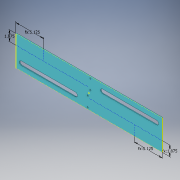
# Autodesk Inventor part: 5.5 x 27 x 1/8 x 3/8
Saved by Autodesk Inventor 2016 (Build 200138000, 138)
## iProperties
Created: 2015-06-18
Part Number: 5.5 x 27 x 1/8 x 3/8
Material: Aluminum 6061
Document SubType Name: Modeling
Designer: steele
Density: 2.7 g/cm^3
Appearance: Cadet Blue
Mass: 732.367 g
Surface Area: 1799.65 cm^2
Volume: 271.247 cm^3
Author: steele
Autodesk Inventor part; units mm, degrees
ref_plane "YZ Plane" through (0, 0, 0) normal (1, 0, 0) x (0, 1, 0)
ref_plane "XZ Plane" through (0, 0, 0) normal (0, 1, 0) x (-1, 0, 0)
ref_plane "XY Plane" through (0, 0, 0) normal (0, 0, 1) x (1, 0, 0)
sketch "Sketch1" plane through (0, 0, 0) normal (1, 0, 0) x (0, 1, 0)
  line L0 (-69.85, 342.9) -> (-69.85, -342.9)
  line L1 (-69.85, -342.9) -> (69.85, -342.9)
  line L2 (69.85, -342.9) -> (69.85, 342.9)
  line L3 (69.85, 342.9) -> (-69.85, 342.9)
  line L4 (-69.85, 342.9) -> (69.85, -342.9) construction
  line L5 (-69.85, -342.9) -> (69.85, 342.9) construction
  point P0 (0, 0)
  dimension "width" = 685.8
  dimension "height" = 139.7
  constraints: 12 end point, 2 midpoint, 2 parallel, 1 perpendicular, 1 vertical
  measures "width" distance of L0.start L0.end
  measures "height" distance of L0.end L1.end
extrude "Extrusion1" add sketch "Sketch1" along normal blind 3.175
sketch "Sketch2" plane through (3.175, 0, 0) normal (1, 0, 0) x (0, 0, -1)
  line L0 (-317.5, 38.1) -> (-63.5, 38.1) construction
  line L1 (-317.5, 28.575) -> (-63.5, 28.575)
  line L2 (-63.5, 47.625) -> (-317.5, 47.625)
  arc A0 (-317.5, 47.625) -> (-317.5, 28.575) centre (-317.5, 38.1) ccw
  arc A1 (-63.5, 28.575) -> (-63.5, 47.625) centre (-63.5, 38.1) ccw
  line L3 (342.9, 69.85) -> (-342.9, 69.85) projected
  line L4 (-342.9, 69.85) -> (-342.9, -69.85) projected
  line L5 (63.5, -38.1) -> (317.5, -38.1) construction
  line L6 (63.5, -47.625) -> (317.5, -47.625)
  line L7 (317.5, -28.575) -> (63.5, -28.575)
  arc A2 (63.5, -28.575) -> (63.5, -47.625) centre (63.5, -38.1) ccw
  arc A3 (317.5, -47.625) -> (317.5, -28.575) centre (317.5, -38.1) ccw
  line L8 (-342.9, -69.85) -> (342.9, -69.85) projected
  line L9 (342.9, -69.85) -> (342.9, 69.85) projected
  point P0 (0, 0)
  point P1 (-190.5, 38.1)
  point P2 (190.5, -38.1)
  dimension "slot_center_from_top" = 31.75
  dimension "slot_center_from_side" = 152.4
  dimension "slot_radius" = 9.525
  dimension "d7" = 31.75
  dimension "d8" = 152.4
  dimension "d9" = 9.525
  dimension "length_of_slot" = 254
  dimension "d13" = 254
  constraints: 16 end point, 8 point on circle, 8 tangent, 4 centre point, 2 horizontal, 2 midpoint, 2 parallel
  measures "slot_center_from_top" distance from line of point (-190.5, 38.1) L3
  measures "slot_center_from_side" distance from line of point (-190.5, 38.1) L4
  measures "slot_radius" radius of A1
  measures "d7" distance from line of point (190.5, -38.1) L8
  measures "d8" distance from line of point (190.5, -38.1) L9
  measures "d9" radius of A2
  measures "length_of_slot" distance of L0.start L0.end
  measures "d13" distance of L5.start L5.end
extrude "Extrusion2" cut sketch "Sketch2" against normal through all contours A0 L2 A1 L1 | A2 L7 A3 L6
sketch "Sketch3" plane through (0, 0, 0) normal (-1, 0, 0) x (0, 0, 1)
  line L0 (-342.9, 69.85) -> (342.9, 69.85) construction
  line L1 (6.3584, 69.85) -> (6.3584, -72.7678) construction
  line L2 (342.9, 69.85) -> (342.9, -69.85) construction
  line L3 (-6.3584, 69.85) -> (-6.3584, -69.85) construction
  line L4 (-342.9, -69.85) -> (-342.9, 69.85) construction
  line L5 (-6.3584, 61.976) -> (6.3584, 61.976) construction
  line L6 (-6.3584, -61.976) -> (6.3584, -61.976) construction
  line L7 (342.9, -69.85) -> (-342.9, -69.85) construction
  line L8 (-6.3584, 14.224) -> (6.3584, 14.224) construction
  line L9 (-6.3584, -14.224) -> (6.3584, -14.224) construction
  point P0 (0, 0)
  point P1 (80.6051, 237.827)
  point P2 (47.886, -92.9067)
  dimension "Vertical_Line_For_Bolt_Holes" = 336.5416
  dimension "d15" = 336.5416
  dimension "First_Horizontal_Line" = 7.874
  dimension "d17" = 7.874
  dimension "Second_Horizontal_Line" = 47.752
  dimension "d19" = 47.752
  constraints: 12 end point, 10 point on line, 6 coincident, 4 perpendicular, 2 vertical
  measures "Vertical_Line_For_Bolt_Holes" distance between parallel lines of L1 L2
  measures "d15" distance between parallel lines of L3 L4
  measures "First_Horizontal_Line" distance between parallel lines of L5 L0
  measures "d17" distance between parallel lines of L7 L6
  measures "Second_Horizontal_Line" distance between parallel lines of L8 L5
  measures "d19" distance from line of point (-6.358, -61.976) L9
hole "Hole1" at (0, 61.976, 6.3584) at (0, -61.976, -6.3584) at (0, 237.827, 80.6051) at (0, -92.9067, 47.886) at (0, 14.224, 6.3584) at (0, -14.224, -6.3584) direction (1, 0, 0) diameter 6.35 end through all
sketch "Sketch4" plane through (0, 0, 0) normal (-1, 0, 0) x (0, 0, 1)
  line L0 (-342.6701, 22.225) -> (0, 22.225) construction
  line L1 (343.1993, -22.225) -> (0, -22.225) construction
  line L2 (-342.9, 69.85) -> (342.9, 69.85) construction
  line L3 (342.9, -69.85) -> (-342.9, -69.85) construction
  line L4 (-342.9, -69.85) -> (-342.9, 69.85) projected
  line L5 (342.9, 69.85) -> (342.9, -69.85) projected
  line L6 (-212.725, 22.225) -> (-212.725, 69.85) construction
  line L7 (-342.9, 69.85) -> (342.9, 69.85) construction
  line L8 (212.725, -22.225) -> (212.725, -69.85) construction
  point P0 (0, 0)
  dimension "horizontalHoleForStopSupport" = 47.625
  dimension "d28" = 47.625
  dimension "d31" = 130.175
  dimension "d32" = 130.175
  constraints: 8 end point, 4 point on line, 2 horizontal, 2 perpendicular
  measures "horizontalHoleForStopSupport" distance between parallel lines of L0 L2
  measures "d28" distance between parallel lines of L3 L1
  measures "d31" distance between parallel lines of L6 L4
  measures "d32" distance between parallel lines of L8 L5
equation "\"d7\" = slot_center_from_top"
equation "\"d8\" = slot_center_from_side"
equation "\"d9\" = slot_radius"
equation "\"d13\" = length_of_slot"
equation "\"d15\" = Vertical_Line_For_Bolt_Holes"
equation "\"d17\" = First_Horizontal_Line"
equation "\"d19\" = Second_Horizontal_Line"
equation "\"d28\" = horizontalHoleForStopSupport"
equation "\"d31\" = verticalDistanceForSupportHole"
equation "\"d32\" = verticalDistanceForSupportHole"
equation "\"verticalDistanceForSupportHole\" = 130.175"
body "Solid1"
